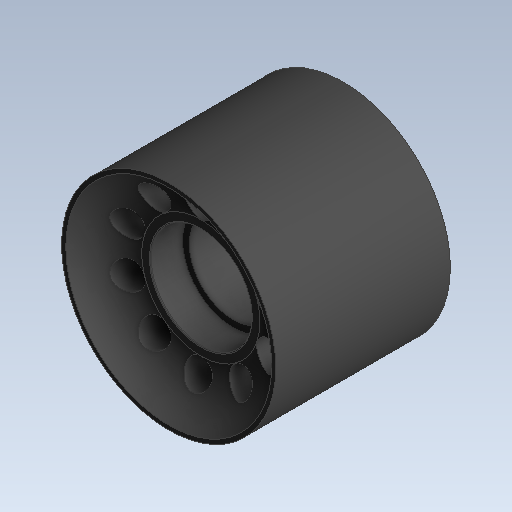
# Autodesk Inventor part: Kegel_core
Saved by Autodesk Inventor 2020.1 (Build 241239000, 239)
## iProperties
Created: 2018-01-15
Part Number: Kegel_core
Material: ABS Plastic
Document SubType Name: Modeling
Designer: Tobias
Density: 1.06 g/cm^3
Appearance: Rubber - Black
Mass: 34.3907 g
Surface Area: 148.554 cm^2
Volume: 32.444 cm^3
Author: Tobias
Autodesk Inventor part; units mm, degrees
ref_plane "YZ Plane" through (0, 0, 0) normal (1, 0, 0) x (0, 1, 0)
ref_plane "XZ Plane" through (0, 0, 0) normal (0, 1, 0) x (-1, 0, 0)
sketch "Sketch1" plane through (0, 0, 0) normal (0, 0, 1) x (1, 0, 0)
  circle A0 centre (0, 0) radius 23.3
  dimension "d15" = 46.6
  constraints: 1 centre point, 1 coincident
  measures "d15" diameter of A0
extrude "Extrusion1" add sketch "Sketch1" along normal mid plane 38
sketch "Sketch2" plane through (0, 0, 0) normal (0, 0, 1) x (1, 0, 0)
  circle A0 centre (0, 0) radius 9.5
  dimension "d2" = 19
  constraints: 1 centre point, 1 coincident
  measures "d2" diameter of A0
extrude "Extrusion2" cut sketch "Sketch2" along normal mid plane 56
sketch "Sketch5" plane through (0, 0, 0) normal (0, 1, 0) x (-1, 0, 0)
  line L0 (0, -6) -> (0, 36) projected
  line L1 (-32.62, 0) -> (32.62, 0) projected
  line L2 (22.4, 30) -> (0, 30)
  line L3 (0, 30) -> (0, 12)
  line L4 (0, 12) -> (22.4, 12)
  line L5 (22.4, 12) -> (22.4, 30)
  point P0 (0, 0)
  dimension "d18" = 30
  dimension "d31" = 44.8
  dimension "d32" = 12
  constraints: 8 end point, 2 parallel, 1 horizontal, 1 perpendicular, 1 point on line
  measures "d18" distance between parallel lines of L1 L2
  measures "d31" diameter of L5 L0
  measures "d32" distance between parallel lines of L4 L1
revolve "Revolution1" cut sketch "Sketch5" angle 360 about axis through (0, 0, 0) along (0, 0, 1)
mirror "Mirror2" about plane through (0, 0, 0) normal (0, 0, 1) of "Revolution1"
fillet "Fillet1" radius 10 2 edges at (22.4, 0, 12) (22.4, 0, -12)
sketch "Sketch4" plane through (0, 0, 0) normal (0, 0, 1) x (1, 0, 0)
  circle A0 centre (0, 0) radius 15.85 construction
  line L0 (0, 25.67) -> (0, -22.77) projected
  line L1 (-22.19, 0) -> (22.19, 0) projected
  circle A1 centre (0, 15.85) radius 2.9
  dimension "d8" = 31.7
  dimension "d9" = 5.8
  constraints: 1 centre point, 1 coincident, 1 point on line, 1 vertical alignment, 2 other
  measures "d9" diameter of A1
extrude "Extrusion4" cut sketch "Sketch4" along normal through all both and the other way through all
pattern_circular "Circular Pattern1" count 10 over 360 about axis through (0, 0, -10) along (0, 0, 1) of "Extrusion4"
ref_plane "Work Plane1" through (0, 0, 5) normal (0, 0, 1) x (1, 0, 0)
sketch "Sketch7" plane through (0, 0, 5) normal (0, 0, 1) x (1, 0, 0)
  circle A0 centre (0, 0) radius 11
  dimension "d34" = 22
  constraints: 1 centre point, 1 coincident
  measures "d34" diameter of A0
extrude "Extrusion5" cut sketch "Sketch7" along normal blind 20
mirror "Mirror3" about plane through (0, 0, 0) normal (0, 0, 1) of "Extrusion5"
fillet "Fillet5" radius 0.2 2 edges at (-11, 0, 12) (-11, 0, -12)
body "Solid1"
